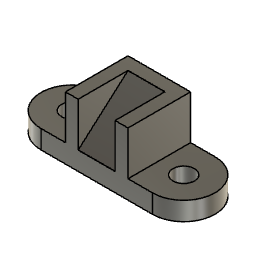
A2 (Autodesk Fusion 360 design; units mm, degrees)
Autodesk Fusion 360 part; units mm, degrees
sketch "Base_Sketch" plane through (0, 0, 0) normal (0, 0, 1) x (1, 0, 0)
  line L0 (57, 32) -> (-57, 32)
  line L1 (-57, -32) -> (57, -32)
  circle A0 centre (-57, 0) radius 11
  circle A1 centre (57, 0) radius 11
  arc A2 (-57, 32) -> (-57, -32) centre (-57, 0) ccw
  arc A3 (57, -32) -> (57, 32) centre (57, 0) ccw
  dimension "d1" = 114
  dimension "d2" = 64
  dimension "d3" = 32
  dimension "d4" = 32
  constraint horizontal L0
  constraint parallel L0 L1
  measures "d1" distance of L1.start L1.end
  measures "d2" distance of L0.end L1.start
  measures "d3" radius of A2
  measures "d4" radius of A3
extrude "Extrude1" add sketch "Base_Sketch" along normal blind 19
sketch "Top_Base_Sketch" plane through (0, 0, 19) normal (0, 0, 1) x (-1, 0, 0)
  circle A0 centre (-57, 0) radius 11
  circle A1 centre (57, 0) radius 11
  arc A2 (-57, 32) -> (-57, -32) centre (-57, 0) ccw
  line L0 (-57, -32) -> (57, -32)
  arc A3 (57, -32) -> (57, 32) centre (57, 0) ccw
  line L1 (57, 32) -> (-57, 32)
  line L2 (32, -32) -> (32, 32)
  line L3 (-32, -32) -> (-32, 32)
  line L4 (19, 32) -> (19, -19)
  line L5 (-18.7586, 32) -> (-18.7586, -19)
  line L6 (19, -19) -> (-19, -19)
  line L7 (32, 32) -> (19, 32) construction
  line L8 (32, -32) -> (-32, -32) construction
  line L9 (-18.7586, 32) -> (-32, 32) construction
  dimension "d9" = 64
  dimension "d11" = 51
  dimension "d12" = 51
  dimension "d13" = 38
  dimension "d15" = 13
  constraint coincident L0 L2.start
  constraint coincident L1 L2.end
  constraint perpendicular L1 L2
  constraint coincident L0 L3.start
  constraint coincident L1 L3.end
  constraint perpendicular L1 L3
  constraint coincident L1 L4.start
  constraint perpendicular L1 L4
  constraint coincident L1 L5.start
  constraint perpendicular L1 L5
  constraint perpendicular L5 L6
  measures "d9" distance of L2 L3
  measures "d11" distance of L4.start L4.end
  measures "d12" distance of L5.start L5.end
  measures "d13" distance of L4.end L6.end
  measures "d15" distance of L2 L4
extrude "Extrude2" add sketch "Top_Base_Sketch" along normal blind 45 contours L0 L1 L2 L3 L4 L5 L6
sketch "Triangle_Sketch" plane through (0, 0, 0) normal (1, 0, 0) x (0, 1, 0)
  line L0 (18.9506, 63.9102) -> (18.9506, 18.9102)
  line L1 (18.9506, 18.9102) -> (-32.0494, 18.9102)
  line L2 (-32.0494, 18.9102) -> (18.9506, 63.9102)
  dimension "d18" = 45
  dimension "d20" = 51
  constraint vertical L0
  constraint perpendicular L0 L1
  measures "d18" distance of L0.start L0.end
  measures "d20" distance of L0.end L1.end
extrude "Extrude3" add sketch "Triangle_Sketch" along normal mid plane 38
named bodies: "A2_Body"
